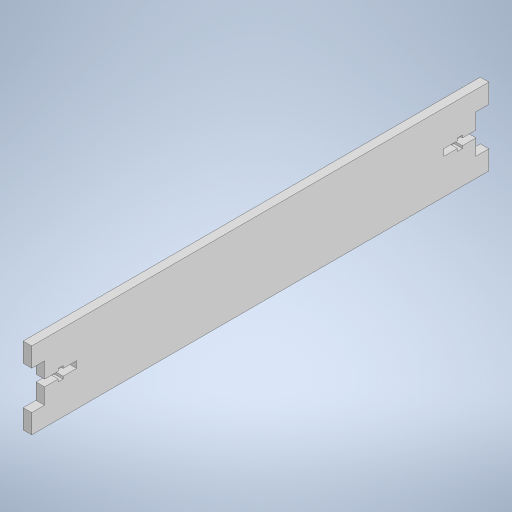
# Autodesk Inventor part: ребро
Saved by Autodesk Inventor 2023.1 (Build 271208000, 208)
## iProperties
Created: 2024-12-25
Part Number: ребро
Material: Типовые
Document SubType Name: Modeling
Designer: DELL
Density: 1 g/cm^3
Appearance: По умолчанию
Author: DELL
Autodesk Inventor part; units mm, degrees
ref_plane "YZ Plane" through (0, 0, 0) normal (1, 0, 0) x (0, 1, 0)
ref_plane "XZ Plane" through (0, 0, 0) normal (0, 1, 0) x (-1, 0, 0)
ref_plane "XY Plane" through (0, 0, 0) normal (0, 0, 1) x (1, 0, 0)
sketch "Эскиз1" plane through (0, 0, 0) normal (0, 0, 1) x (1, 0, 0)
  line L0 (-2, 18) -> (2, 18)
  line L1 (2, -18) -> (-2, -18)
  line L2 (-2, 18) -> (2, -18) construction
  line L3 (2, 18) -> (-2, -18) construction
  line L4 (-2, 9) -> (2, 9)
  line L5 (2, -9) -> (-2, -9)
  line L6 (-2, 9) -> (2, -9) construction
  line L7 (2, 9) -> (-2, -9) construction
  line L8 (-2, -18) -> (-2, -9)
  line L9 (-2, 9) -> (-2, 18)
  line L10 (2, 18) -> (2, 9)
  line L11 (2, -9) -> (2, -18)
  point P0 (0, 0)
  dimension "d4" = 36
  dimension "d5" = 4
  constraints: 24 end point, 6 parallel, 4 midpoint, 2 horizontal, 2 perpendicular
  measures "d4" distance of L1.start L0.end
  measures "d5" distance of L4.start L4.end
extrude "Выдавливание1" add sketch "Эскиз1" along normal blind 6
sketch "Эскиз2" plane through (0, 0, 6) normal (0, 0, 1) x (1, 0, 0)
  line L0 (-2, -18) -> (2, -18) projected
  line L1 (2, 18) -> (-2, 18) projected
  line L2 (-2, -18) -> (2, -18)
  line L3 (2, -18) -> (2, 18)
  line L4 (2, 18) -> (-2, 18)
  line L5 (-2, 18) -> (-2, -18)
  point P0 (0, 0)
  constraints: 8 end point, 2 parallel, 1 horizontal, 1 perpendicular
extrude "Выдавливание2" add sketch "Эскиз2" along normal blind 201.8
sketch "Эскиз4" plane through (0, 0, 207.8) normal (0, 0, 1) x (1, 0, 0)
  line L0 (2, 18) -> (-2, 18) projected
  line L1 (-2, -18) -> (2, -18) projected
  line L2 (-2, 18) -> (2, 18)
  line L3 (2, -18) -> (-2, -18)
  line L4 (-2, 9) -> (-2, -9) projected
  line L5 (2, 9) -> (-2, 9)
  line L6 (-2, -9) -> (2, -9)
  line L7 (2, 9) -> (-2, -9) construction
  line L8 (-2, 9) -> (2, -9) construction
  line L9 (2, 18) -> (2, 9)
  line L10 (2, -9) -> (2, -18)
  line L11 (-2, -18) -> (-2, -9)
  line L12 (-2, 9) -> (-2, 18)
  point P0 (0, 0)
  constraints: 20 end point, 6 parallel, 2 horizontal, 2 midpoint, 2 perpendicular
extrude "Выдавливание3" add sketch "Эскиз4" along normal blind 6
sketch "Эскиз5" plane through (-2, -18, 0) normal (-1, 0, 0) x (0, 0, 1)
  line L0 (106.9, -127.9343) -> (106.9, 327.3325) construction
  line L1 (207.8, 27) -> (207.8, 9) projected
  line L2 (192.8, 19.575) -> (192.8, 16.425)
  line L3 (207.8, 16.425) -> (207.8, 19.575)
  line L4 (207.8, 19.575) -> (192.8, 16.425) construction
  line L5 (192.8, 19.575) -> (207.8, 16.425) construction
  line L6 (201.45, 15.25) -> (199.15, 15.25)
  line L7 (199.15, 20.75) -> (201.45, 20.75)
  line L8 (201.45, 15.25) -> (199.15, 20.75) construction
  line L9 (199.15, 15.25) -> (201.45, 20.75) construction
  line L10 (201.45, 20.75) -> (201.45, 19.575)
  line L11 (201.45, 16.425) -> (201.45, 15.25)
  line L12 (207.8, 19.575) -> (201.45, 19.575)
  line L13 (199.15, 19.575) -> (192.8, 19.575)
  line L14 (192.8, 16.425) -> (199.15, 16.425)
  line L15 (201.45, 16.425) -> (207.8, 16.425)
  line L16 (199.15, 15.25) -> (199.15, 16.425)
  line L17 (199.15, 19.575) -> (199.15, 20.75)
  line L18 (6, 27) -> (6, 9)
  line L19 (21, 19.575) -> (21, 16.425)
  line L20 (6, 16.425) -> (6, 19.575)
  line L21 (6, 19.575) -> (21, 16.425) construction
  line L22 (21, 19.575) -> (6, 16.425) construction
  line L23 (12.35, 15.25) -> (14.65, 15.25)
  line L24 (14.65, 20.75) -> (12.35, 20.75)
  line L25 (12.35, 15.25) -> (14.65, 20.75) construction
  line L26 (14.65, 15.25) -> (12.35, 20.75) construction
  line L27 (12.35, 20.75) -> (12.35, 19.575)
  line L28 (12.35, 16.425) -> (12.35, 15.25)
  line L29 (6, 19.575) -> (12.35, 19.575)
  line L30 (14.65, 19.575) -> (21, 19.575)
  line L31 (21, 16.425) -> (14.65, 16.425)
  line L32 (12.35, 16.425) -> (6, 16.425)
  line L33 (14.65, 15.25) -> (14.65, 16.425)
  line L34 (14.65, 19.575) -> (14.65, 20.75)
  point P0 (6, 27)
  point P1 (6, 9)
  point P2 (200.3, 18)
  point P3 (207.8, 18)
  point P4 (13.5, 18)
  point P5 (6, 18)
  point P6 (207.8, 19.575)
  dimension "d25" = 15
  dimension "d26" = 3.15
  dimension "d27" = 2.3
  dimension "d28" = 5.5
  constraints: 68 end point, 16 symmetric about line, 10 parallel, 6 midpoint, 4 perpendicular, 3 horizontal, 1 vertical
  measures "d25" distance of L2.end L3.start
  measures "d26" distance of L2.start L2.end
  measures "d27" distance of L7.start L7.end
  measures "d28" distance of L6.end L7.start
extrude "Выдавливание4" cut sketch "Эскиз5" against normal blind 6
